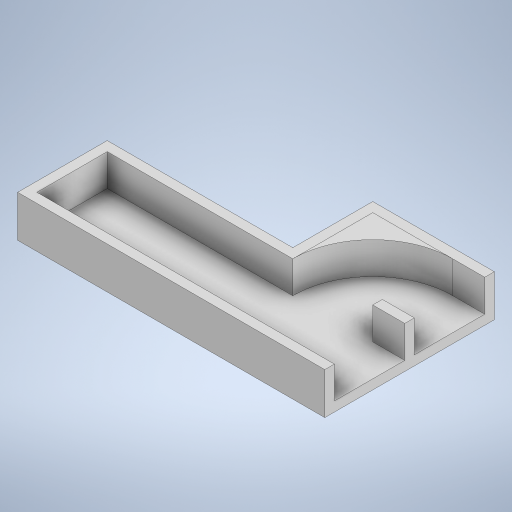
# Autodesk Inventor part: Trilho 5 min
Saved by Autodesk Inventor 2024 (Build 280153000, 153)
## iProperties
Created: 2023-05-22
Part Number: Trilho 5 min
Material: Genérico
Document SubType Name: Modeling
Designer: jpjoa
Density: 1 g/cm^3
Appearance: Padrão
Author: jpjoa
Autodesk Inventor part; units mm, degrees
ref_plane "YZ Plane" through (0, 0, 0) normal (1, 0, 0) x (0, 1, 0)
ref_plane "XZ Plane" through (0, 0, 0) normal (0, 1, 0) x (-1, 0, 0)
ref_plane "XY Plane" through (0, 0, 0) normal (0, 0, 1) x (1, 0, 0)
sketch "Esboço1" plane through (0, 0, 0) normal (0, 1, 0) x (-1, 0, 0)
  line L0 (-93, -3) -> (0, -3)
  line L1 (0, -25) -> (-58, -25)
  line L2 (-93, 0) -> (-93, -28)
  line L3 (-93, -28) -> (-83, -28)
  line L4 (-55, -28) -> (0, -28)
  line L5 (0, -28) -> (0, 0)
  line L6 (0, 0) -> (-93, 0)
  line L7 (-55, -28) -> (-55, -53)
  line L8 (-55, -53) -> (-93, -53)
  line L9 (-93, -53) -> (-93, -50)
  line L10 (-93, -50) -> (-58, -50)
  line L11 (-58, -50) -> (-58, -25)
  arc A0 (-83, -50) -> (-58, -25) centre (-83, -25) ccw
  arc A1 (-83, -28) -> (-80, -25) centre (-83, -25) ccw
  line L12 (-93, -25) -> (-80, -25)
  line L13 (0, 0) -> (3, 0)
  line L14 (3, 0) -> (3, -28)
  line L15 (3, -28) -> (0, -28)
  line L16 (-83, -28) -> (-83, -25)
  line L17 (-93, -50) -> (-93, -28)
  point P0 (-93, -14)
  point P1 (-93, -51.5)
  point P2 (-83, -28)
  dimension "d7" = 22
  dimension "d9" = 3
  dimension "d10" = 3
  dimension "d13" = 3
  dimension "d14" = 3
  dimension "d16" = 22
  dimension "d20" = 22
  dimension "d21" = 80
  dimension "d29" = 3
  dimension "d31" = 10
  constraints: 36 end point, 8 perpendicular, 5 point on line, 4 horizontal, 4 point on circle, 3 horizontal alignment, 2 centre point, 2 coincident, 2 midpoint, 2 vertical, 2 vertical alignment, 1 collinear
  measures "d7" distance between parallel lines of L0 L1
  measures "d9" distance between parallel lines of L1 L4
  measures "d10" distance between parallel lines of L6 L0
  measures "d13" distance between parallel lines of L11 L7
  measures "d14" distance between parallel lines of L10 L8
  measures "d16" distance between parallel lines of L10 L4
  measures "d20" radial gap between concentric circles of A0 A1
  measures "d21" distance from line of L5 L12.end
  measures "d29" distance between parallel lines of L14 L5
  measures "d31" distance of L9.end A0.start
extrude "Extrusão1" add sketch "Esboço1" against normal blind 3
extrude "Extrusão2" add sketch "Esboço1" along normal blind 10 contours L2 L6 L5 L0 | L5 L13 L14 L15 | L12 L16 L3 L2 | L5 L4 L7 L8 L9 L10 L11 L1
extrude "Extrusão3" add sketch "Esboço1" along normal blind 10 separate body contours L11 L10 A0
equation "\"d9\" = mdf"
equation "\"d10\" = mdf"
equation "\"d13\" = mdf"
equation "\"d14\" = mdf"
equation "\"mdf\" = 3"
equation "\"margem\" = 1"
